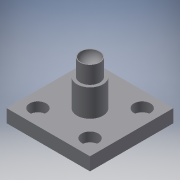
# Autodesk Inventor part: 9mm_holder_MM_9-68_diameter_Original
Saved by Autodesk Inventor 2017 (Build 210142000, 142)
## iProperties
Created: 2008-05-07
Part Number: 9mm_holder_MM_9-68_diameter_Original
Document SubType Name: Modeling
Designer: osbornej
Density: 1 g/cm^3
Mass: 5.78507 g
Surface Area: 32.2527 cm^2
Volume: 5.78507 cm^3
Material: Generic
Appearance: Default
Author: osbornej
Autodesk Inventor part; units mm, degrees
ref_plane "YZ Plane" through (0, 0, 0) normal (1, 0, 0) x (0, 1, 0)
ref_plane "XZ Plane" through (0, 0, 0) normal (0, 1, 0) x (-1, 0, 0)
ref_plane "XY Plane" through (0, 0, 0) normal (0, 0, 1) x (1, 0, 0)
sketch "Sketch1" plane through (0, 0, 0) normal (0, 0, 1) x (1, 0, 0)
  line L0 (0.2333, 13.7206) -> (1.7438, 13.7206)
  line L1 (6.5833, -5.8539) -> (0.2333, -5.8539)
  line L2 (0.2333, -5.8539) -> (0.2333, 13.7206)
  line L3 (1.7438, 13.7206) -> (1.7438, 22.1437)
  line L4 (1.7438, 22.1437) -> (2.1004, 22.1437)
  line L5 (6.5833, 18.0359) -> (6.5833, -5.8539)
  arc A0 (2.1004, 22.1437) -> (6.5833, 18.0359) centre (6.5833, 22.5359) ccw
  line L6 (6.5833, 22.5359) -> (2.1004, 22.1437) construction
  line L7 (6.5833, 22.5359) -> (6.5833, 18.0359) construction
  dimension "d131" = 6.35
  dimension "d136" = 4.5
  dimension "d137" = 85
  constraints: 16 end point, 3 parallel, 2 perpendicular, 2 point on circle, 1 centre point, 1 horizontal, 1 vertical
  measures "d131" distance between parallel lines of L5 L2
  measures "d136" radius of A0
  measures "d137" angle of L6 L7
revolve "Revolution1" add sketch "Sketch1" angle 360 about axis through (6.5833, 18.0359, 0) along (0, -1, 0)
ref_plane "Work Plane1" through (0.2333, -5.8539, 0) normal (-1, 0, 0) x (0, -1, 0)
hole "Hole7" at (6.5833, -5.8539, 0) direction (0, 1, 0) diameter 7.9502 depth 12.7 tip angle 118 taper from width 8.7311 to width 8.3566 over 5.9944 thread size "1/8" designation "1/8 - 27 NPT" standard "NPT for PVC Pipe and Fitting"
hole "Hole8" at (6.5833, -5.8539, 0) direction (0, 1, 0) diameter 3.175 depth 20.32 tip angle 118
hole "Hole9" at (6.5833, 22.1437, 0) direction (0, -1, 0) diameter 1.016 end through all
hole "Hole10" at (6.5833, 22.1437, 0) direction (0, -1, 0) diameter 1.5748 depth 12.7 tip angle 118
sketch "Sketch4" plane through (6.5833, -5.8539, 0) normal (0, -1, 0) x (1, 0, 0)
  line L0 (20.32, 20.32) -> (-20.32, 20.32)
  line L1 (-20.32, 20.32) -> (-20.32, -20.32)
  line L2 (-20.32, -20.32) -> (20.32, -20.32)
  line L3 (20.32, -20.32) -> (20.32, 20.32)
  circle A0 centre (0, 0) radius 6.35 projected
  line L4 (20.32, 20.32) -> (-20.32, -20.32) construction
  line L5 (-20.32, 20.32) -> (20.32, -20.32) construction
  point P0 (-6.5833, 0)
  point P1 (12.6896, -12.6896)
  point P2 (12.6896, 12.6896)
  point P3 (-12.6896, 12.6896)
  point P4 (-12.6896, -12.6896)
  dimension "d115" = 40.64
  dimension "d116" = 40.64
  constraints: 12 end point, 4 point on line, 2 midpoint, 2 parallel, 1 horizontal, 1 perpendicular
  measures "d115" distance of L2.end L1.end
  measures "d116" distance of L0.end L1.end
extrude "Extrusion3" add sketch "Sketch4" against normal blind 6.35
sketch "Sketch8" plane through (6.5833, 0.4961, 0) normal (0, 1, 0) x (1, 0, 0)
  point P0 (-6.5833, 0)
  point P1 (-12.6698, 12.6961)
  point P2 (12.7223, 12.6961)
  point P3 (12.7223, -12.6961)
  point P4 (-12.6698, -12.6961)
hole "Hole11" at (-6.0865, 0.4961, -12.6961) at (19.3056, 0.4961, -12.6961) at (19.3056, 0.4961, 12.6961) at (-6.0865, 0.4961, 12.6961) direction (0, -1, 0) diameter 4.9784 end through all counterbore diameter 8.0772 counterbore depth 4.572
body "Solid1"
